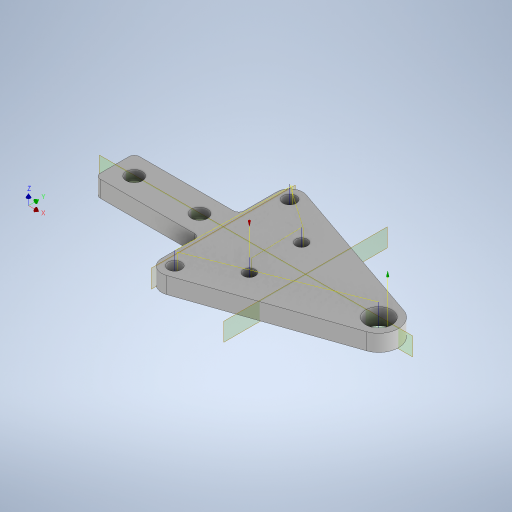
# Autodesk Inventor part: XZ Plate
Saved by Autodesk Inventor 2023.1 (Build 271208000, 208)
## iProperties
Created: 2022-10-29
Part Number: XZ Plate
Material: Generic
Document SubType Name: Modeling
Designer: nicol
Density: 1 g/cm^3
Appearance: Default
Author: nicol
Autodesk Inventor part; units mm, degrees
ref_plane "XY Plane" through (0, 0, 0) normal (0, 0, 1) x (1, 0, 0)
sketch "Sketch1" plane through (0, 0, 0) normal (0, 0, 1) x (1, 0, 0)
  line L0 (-20, 150) -> (20, 150) construction
  line L1 (20, 150) -> (20, -150) construction
  line L2 (20, -150) -> (-20, -150) construction
  line L3 (-20, -150) -> (-20, 150) construction
  circle A0 centre (-28.08, 22) radius 10.72 construction
  circle A1 centre (-28.08, -22) radius 10.72 construction
  circle A2 centre (28.08, 0) radius 10.72 construction
  line L4 (38.8, 4.056) -> (38.8, -13.1126) construction
  circle A3 centre (28.08, 0) radius 7.5
  circle A4 centre (-28.08, 22) radius 5
  circle A5 centre (-28.08, -22) radius 5
  line L5 (-33.08, 3.8118) -> (-33.08, -3.8118) construction
  line L6 (0, 150) -> (0, -150) construction
  line L7 (-20, -108) -> (-20, -150) construction
  line L8 (-20, 150) -> (-20, 108) construction
  line L9 (-73.08, 7.5) -> (-33.08, 7.5)
  line L10 (-33.08, 7.5) -> (-33.08, -7.5)
  line L11 (-33.08, -7.5) -> (-73.08, -7.5)
  line L12 (-73.08, -7.5) -> (-73.08, 7.5)
  circle A6 centre (0, -150) radius 6 construction
  circle A7 centre (-11.5, -10) radius 4.5
  circle A8 centre (0, -150) radius 7
  line L13 (-7, -150) -> (-7, -10)
  line L14 (-11.5, 5.5) -> (-177.58, 5.5)
  line L15 (-11.5, -5.5) -> (-177.58, -5.5)
  line L16 (-183.08, -10) -> (-33.08, -10) construction
  line L17 (-33.08, -10) -> (-33.08, 10) construction
  line L18 (-33.08, 10) -> (-183.08, 10) construction
  line L19 (-183.08, 10) -> (-183.08, -10) construction
  circle A9 centre (-177.58, 0) radius 4.5 construction
  circle A10 centre (-177.58, 0) radius 5.5
  circle A11 centre (-11.5, -10) radius 2.5 construction
  line L20 (-33.08, -22) -> (-33.08, 22)
  line L21 (-26.4508, -26.7271) -> (30.5238, -7.0907)
  line L22 (-26.4508, 26.7271) -> (30.5238, 7.0907)
  line L23 (-20, 0) -> (0, 0)
  circle A12 centre (0, 150) radius 4.5 construction
  circle A13 centre (0, 150) radius 7
  line L24 (-7, 150) -> (-7, 10)
  circle A14 centre (-11.5, 10) radius 4.5
  line L25 (7, -150) -> (7, 150)
  point P0 (20, 0)
  point P1 (-29.8, 0)
  point P2 (-33.0748, -21.7719)
  point P3 (-33.0748, 21.7719)
  point P4 (-26.0808, 26.5829)
  point P5 (30.2394, 7.1824)
  point P6 (30.2394, -7.1824)
  point P7 (-26.0808, -26.5829)
  point P8 (-33.08, 0)
  point P9 (-65.58, 0)
  point P10 (-40.58, 0)
  point P11 (-73.08, 0)
  point P12 (-33.08, 0)
  point P13 (-94.54, -5.5)
  point P14 (-183.08, 0)
  dimension "d0" = 40
  dimension "d1" = 300
  dimension "d2" = 21.44
  dimension "d3" = 22
  dimension "d4" = 22
  dimension "d5" = 58.8
  dimension "d6" = 28.08
  dimension "d7" = 28.08
  dimension "d12" = 15
  dimension "d38" = 10
  dimension "d42" = 15
  dimension "d43" = 40
  dimension "d44" = 25
  dimension "d45" = 7.5
  dimension "d46" = 7.5
  dimension "d48" = 12
  dimension "d49" = 9
  dimension "d51" = 1
  dimension "d53" = 20
  dimension "d55" = 9
  dimension "d56" = 1
  dimension "d60" = 150
  dimension "d74" = 9
  dimension "d75" = 2.5
  dimension "d76" = 9
  constraints: 52 end point, 20 point on circle, 16 tangent, 14 centre point, 11 midpoint, 9 horizontal alignment, 7 parallel, 6 horizontal, 5 vertical, 4 collinear, 3 coincident, 3 equal radius, 3 perpendicular, 3 vertical alignment, 2 other
  measures "d0" distance of L0.start L0.end
  measures "d1" distance of L0.end L1.end
  measures "d2" diameter of A2
  measures "d3" vertical distance of L23.end A1.centre
  measures "d4" vertical distance of A0.centre L23.end
  measures "d5" distance between parallel lines of L3 L4
  measures "d6" distance of A2.centre L23.end
  measures "d7" horizontal distance of L23.end A0.centre
  measures "d12" diameter of A3
  measures "d38" diameter of A4
  measures "d42" distance of L11.end L9.start
  measures "d43" distance of L9.start L9.end
  measures "d44" distance of point (-40.58, 0) point (-65.58, 0)
  measures "d45" distance from line of L5 point (-40.58, 0)
  measures "d46" distance from line of L12 point (-65.58, 0)
  measures "d48" diameter of A6
  measures "d49" diameter of A7
  measures "d53" distance of L18.end L16.start
  measures "d55" diameter of A9
  measures "d56" radial gap between concentric circles of A9 A10
  measures "d60" distance of L17.end L18.end
  measures "d74" diameter of A12
  measures "d75" radial gap between concentric circles of A12 A13
  measures "d76" diameter of A14
extrude "Extrusion1" add sketch "Sketch1" against normal blind 6.35 contours A3 | A3 L21 L25 L22 | L25 L21 L13 A7 L15 L10 L14 A14 L24 L22 | L24 A14 L14 L10 L20 A4 L22 | L21 A5 L20 L10 L15 A7 L13 | A4 | A14 | A7 | A5 | L10 L14 L12 L9 | L10 L15 L12 L14 | L10 L11 L12 L15
hole "Hole1" at (-28.08, 22, 0) at (-28.08, -22, 0) direction (0, 0, -1) diameter 5.1 end through all
hole "Hole2" at (-40.58, 0, 0) at (-65.58, 0, 0) direction (0, 0, -1) diameter 3.2 end through all counterbore diameter 6.2 counterbore depth 3.58
hole "Hole3" at (28.08, 0, 0) direction (0, 0, -1) diameter 10 end through all
ref_plane "Work Plane2" through (-31.4975, 0, 0) normal (1, 0, 0) x (0, 1, 0)
ref_plane "Work Plane3" through (0, 150, 0) normal (-1, 0, 0) x (0, -1, 0)
fillet "Fillet1" radius 2 4 edges at (-73.08, 7.5, -3.175) (-73.08, -7.5, -3.175) (-33.08, -7.5, -3.175) (-33.08, 7.5, -3.175)
hole "Hole4" at (-11.5, -10, 0) at (-11.5, 10, 0) direction (0, 0, -1) diameter 4.5 end through all
sketch "Sketch3" plane through (0, 0, 0) normal (0, 0, 1) x (1, 0, 0)
  circle A0 centre (-11.5, -10) radius 2.25 projected
  circle A1 centre (-11.5, 10) radius 2.25 projected
  circle A2 centre (28.08, 0) radius 5 projected
  circle A3 centre (-40.58, 0) radius 3.1 projected
  circle A4 centre (-65.58, 0) radius 3.1 projected
  circle A5 centre (-28.08, 22) radius 2.55 projected
  circle A6 centre (-28.08, -22) radius 2.55 projected
  arc A7 (-73.08, -5.5) -> (-71.08, -7.5) centre (-71.08, -5.5) ccw projected
  line L0 (-71.08, -7.5) -> (-35.08, -7.5) projected
  arc A8 (-33.08, -9.5) -> (-35.08, -7.5) centre (-35.08, -9.5) ccw projected
  line L1 (-33.08, -9.5) -> (-33.08, -22) projected
  arc A9 (-33.08, -22) -> (-26.4508, -26.7271) centre (-28.08, -22) ccw projected
  line L2 (-26.4508, -26.7271) -> (30.5238, -7.0907) projected
  arc A10 (30.5238, -7.0907) -> (30.5238, 7.0907) centre (28.08, 0) ccw projected
  line L3 (30.5238, 7.0907) -> (-26.4508, 26.7271) projected
  arc A11 (-26.4508, 26.7271) -> (-33.08, 22) centre (-28.08, 22) ccw projected
  line L4 (-33.08, 22) -> (-33.08, 9.5) projected
  arc A12 (-35.08, 7.5) -> (-33.08, 9.5) centre (-35.08, 9.5) ccw projected
  line L5 (-35.08, 7.5) -> (-71.08, 7.5) projected
  arc A13 (-71.08, 7.5) -> (-73.08, 5.5) centre (-71.08, 5.5) ccw projected
  line L6 (-73.08, 5.5) -> (-73.08, -5.5) projected
  point P0 (0, 0)
  constraints: 1 coincident
equation "\"d4\" = d3"
equation "\"d7\" = d6"
equation "\"d46\" = d45"
equation "\"CAM_OFFSET\" = -0.508"
body "Solid1"
